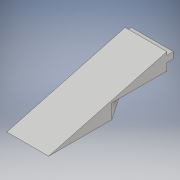
# Autodesk Inventor part: RAMP
Saved by Autodesk Inventor 2017 (Build 210142000, 142)
## iProperties
Created: 2017-03-09
Part Number: RAMP
Material: Generic
Document SubType Name: Modeling
Designer: vitor
Density: 1 g/cm^3
Appearance: Default
Author: vitor
Autodesk Inventor part; units mm, degrees
ref_plane "YZ Plane" through (0, 0, 0) normal (1, 0, 0) x (0, 1, 0)
ref_plane "XZ Plane" through (0, 0, 0) normal (0, 1, 0) x (-1, 0, 0)
ref_plane "XY Plane" through (0, 0, 0) normal (0, 0, 1) x (1, 0, 0)
sketch "Sketch1" plane through (0, 0, 0) normal (1, 0, 0) x (0, 1, 0)
  line L0 (0, 0) -> (24, 0)
  line L1 (24, 0) -> (0, 89.5692)
  line L2 (0, 89.5692) -> (0, 0)
  line L3 (24, 0) -> (30, 0)
  line L4 (7.8518, 60.2659) -> (13.6473, 61.8188)
  line L5 (30, 0) -> (0, 113.0916)
  line L6 (0, 113.0916) -> (0, 89.5692)
  point P0 (0, 23.8051)
  point P1 (17.3305, 0)
  point P2 (0, 30.632)
  dimension "d0" = 24
  dimension "d1" = 75
  dimension "d2" = 6
  dimension "d3" = 6
  dimension "d4" = 90
  constraints: 14 end point, 4 point on line, 2 horizontal, 1 perpendicular, 1 vertical
  measures "d0" distance of L0.start L0.end
  measures "d1" angle of L1 L0
  measures "d2" distance of L0.end L3.end
  measures "d3" distance of L4.start L4.end
  measures "d4" angle of L1 L4
extrude "Extrusion1" add sketch "Sketch1" along normal blind 40
sketch "Sketch5" plane through (0, 0, 0) normal (0, 0, -1) x (-1, 0, 0)
  line L0 (0, 0) -> (0, 30) projected
  line L1 (-40, 0) -> (-4, 0)
  line L2 (-4, 0) -> (-4, 14)
  line L3 (-4, 14) -> (-40, 14)
  line L4 (-40, 14) -> (-40, 0)
  point P0 (0, 18)
  dimension "d24" = 36
  dimension "d25" = 14
  constraints: 8 end point, 2 parallel, 1 horizontal, 1 perpendicular, 1 point on line
  measures "d24" distance of L3.end L2.end
  measures "d25" distance of L2.end L1.end
extrude "Extrusion2" cut sketch "Sketch5" against normal blind 52.575
sketch "Sketch7" plane through (4, 14, 0) normal (0, -1, 0) x (1, 0, 0)
  line L0 (0, 0) -> (0, 52.575) projected
  line L1 (36, 52.575) -> (0, 0)
  line L2 (0, 0) -> (0, 3.8616)
  line L3 (0, 3.8616) -> (33.3558, 52.575)
  line L4 (36, 52.575) -> (0, 52.575) projected
  line L5 (33.3558, 52.575) -> (36, 52.575)
  point P0 (-4, 0)
  constraints: 8 end point, 2 point on line, 1 horizontal
extrude "Extrusion4" add sketch "Sketch7" along normal blind 14 contours L0 L3 L4 L1
sketch "Sketch8" plane through (0, 0, 0) normal (0, -1, 0) x (1, 0, 0)
  line L0 (36.9948, 58.9837) -> (3.2686, 58.9837)
  line L1 (3.2686, 58.9837) -> (3.2686, 93.3042)
  line L2 (3.2686, 93.3042) -> (36.9948, 93.3042)
  line L3 (36.9948, 93.3042) -> (36.9948, 58.9837)
  point P0 (0, 0)
  constraints: 8 end point, 2 parallel, 1 horizontal, 1 perpendicular
extrude "Extrusion5" cut sketch "Sketch8" against normal blind 3.4625
sketch "Sketch9" plane through (0, 3.4625, 0) normal (0, -1, 0) x (1, 0, 0)
  line L0 (36.9948, 58.9837) -> (3.2686, 58.9837) projected
  line L1 (3.2686, 58.9837) -> (3.2686, 93.3042) projected
  line L2 (36.9948, 58.9837) -> (3.2686, 58.9837)
  line L3 (3.2686, 58.9837) -> (3.2686, 72.9495)
  line L4 (3.2686, 72.9495) -> (36.9948, 72.9495)
  line L5 (36.9948, 72.9495) -> (36.9948, 58.9837)
  point P0 (0, 0)
  constraints: 8 end point, 2 parallel, 1 horizontal, 1 perpendicular, 1 point on line
extrude "Extrusion6" cut sketch "Sketch9" against normal blind 6.0625
sketch "Sketch10" plane through (0, 0, 0) normal (0, 0, -1) x (-1, 0, 0)
  line L0 (-40, 30) -> (-40, 0) projected
  line L1 (0, 30) -> (0, 0) projected
  line L2 (-40, 27) -> (0, 27)
  line L3 (0, 27) -> (0, 21)
  line L4 (0, 21) -> (-40, 21)
  line L5 (-40, 21) -> (-40, 27)
  line L6 (0, 30) -> (-40, 30) projected
  dimension "d35" = 6
  dimension "d36" = 3
  constraints: 8 end point, 2 parallel, 2 point on line, 1 horizontal, 1 perpendicular
  measures "d35" distance of L2.end L3.end
  measures "d36" distance between parallel lines of L2 L6
extrude "Extrusion7" add sketch "Sketch10" along normal blind 6 contours L2 L1 L4 L0
body "Solid1"
